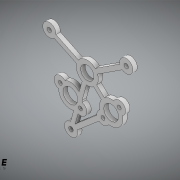
# Autodesk Inventor part: モーターマウントっぽい
Saved by Autodesk Inventor 2020 (Build 240168000, 168)
## iProperties
Created: 2020-01-28
Part Number: モーターマウントっぽい
Material: 一般
Document SubType Name: Modeling
Designer: tanjihayato
Density: 1 g/cm^3
Appearance: 既定
Author: tanjihayato
Autodesk Inventor part; units mm, degrees
ref_plane "YZ Plane" through (0, 0, 0) normal (1, 0, 0) x (0, 1, 0)
ref_plane "XZ Plane" through (0, 0, 0) normal (0, 1, 0) x (-1, 0, 0)
ref_plane "XY Plane" through (0, 0, 0) normal (0, 0, 1) x (1, 0, 0)
sketch "スケッチ1" plane through (0, 0, 0) normal (0, 0, 1) x (1, 0, 0)
  circle A0 centre (16.245, -15.3385) radius 5
  circle A1 centre (21.7373, -9.5217) radius 1.3
  circle A2 centre (10.7528, -21.1553) radius 1.3
  circle A3 centre (-4.6327, -23.2746) radius 1.3
  circle A4 centre (-11.4931, -19.1593) radius 5
  circle A5 centre (-18.3534, -15.044) radius 1.3
  circle A6 centre (26.4774, 17.2466) radius 1.5
  circle A7 centre (-11.0721, -38.6885) radius 1.5
  circle A8 centre (-25.8354, 12.3344) radius 1.5
  circle A9 centre (-11.4931, -19.1593) radius 8
  circle A10 centre (-4.6327, -23.2746) radius 4.3
  circle A11 centre (10.7528, -21.1553) radius 4.3
  circle A12 centre (16.245, -15.3385) radius 8
  circle A13 centre (21.7373, -9.5217) radius 4.3
  circle A14 centre (26.4774, 17.2466) radius 4.5
  circle A15 centre (-25.8354, 12.3344) radius 4.5
  circle A16 centre (-11.0721, -38.6885) radius 4.5
  circle A17 centre (-18.3534, -15.044) radius 4.3
  circle A18 centre (0, 0) radius 4.5
  circle A19 centre (0, 0) radius 7.5
  line L0 (-25.8354, 12.3344) -> (0, 0) construction
  line L1 (-26.4817, 10.9807) -> (-0.6463, -1.3536)
  line L2 (0.6463, 1.3536) -> (-25.1892, 13.688)
  arc A20 (-25.1892, 13.688) -> (-26.4817, 10.9807) centre (-25.8354, 12.3344) ccw
  arc A21 (-0.6463, -1.3536) -> (0.6463, 1.3536) centre (0, 0) ccw
  line L3 (26.4774, 17.2466) -> (0, 0) construction
  line L4 (25.6587, 18.5034) -> (-0.8187, 1.2569)
  line L5 (0.8187, -1.2569) -> (27.2961, 15.9897)
  arc A22 (27.2961, 15.9897) -> (25.6587, 18.5034) centre (26.4774, 17.2466) ccw
  arc A23 (-0.8187, 1.2569) -> (0.8187, -1.2569) centre (0, 0) ccw
  line L6 (0, 0) -> (-11.0721, -38.6885) construction
  line L7 (-1.4421, 0.4127) -> (-12.5142, -38.2758)
  line L8 (-9.63, -39.1013) -> (1.4421, -0.4127)
  arc A24 (1.4421, -0.4127) -> (-1.4421, 0.4127) centre (0, 0) ccw
  arc A25 (-12.5142, -38.2758) -> (-9.63, -39.1013) centre (-11.0721, -38.6885) ccw
  line L9 (0, 0) -> (16.245, -15.3385) construction
  line L10 (-1.0298, -1.0907) -> (15.2152, -16.4292)
  line L11 (17.2748, -14.2479) -> (1.0298, 1.0907)
  arc A26 (1.0298, 1.0907) -> (-1.0298, -1.0907) centre (0, 0) ccw
  arc A27 (15.2152, -16.4292) -> (17.2748, -14.2479) centre (16.245, -15.3385) ccw
  line L12 (16.245, -15.3385) -> (-11.0721, -38.6885) construction
  line L13 (15.2704, -14.1983) -> (-12.0467, -37.5483)
  line L14 (-10.0975, -39.8288) -> (17.2197, -16.4787)
  arc A28 (17.2197, -16.4787) -> (15.2704, -14.1983) centre (16.245, -15.3385) ccw
  arc A29 (-12.0467, -37.5483) -> (-10.0975, -39.8288) centre (-11.0721, -38.6885) ccw
  point P0 (-12.9177, 6.1672)
  point P1 (13.2387, 8.6233)
  point P2 (-5.5361, -19.3443)
  point P3 (8.1225, -7.6693)
  point P4 (2.5865, -27.0135)
  point P5 (17.9324, -7.5185)
  point P6 (11.5612, -8.853)
  point P7 (6.3729, -3.9543)
  point P8 (6.9761, 2.7539)
  point P9 (23.7411, 13.6741)
  point P10 (22.1037, 16.1878)
  point P11 (5.3387, 5.2676)
  point P12 (-5.9852, 4.5196)
  point P13 (-21.3605, 11.8601)
  point P14 (-22.653, 9.1528)
  point P15 (-7.2777, 1.8124)
  point P16 (-3.464, -6.6521)
  point P17 (-5.5202, -13.8372)
  point P18 (-15.2318, -12.0867)
  point P19 (-19.493, -19.1903)
  point P20 (-9.2402, -26.8356)
  point P21 (-11.3469, -34.1969)
  point P22 (-6.8724, -37.0721)
  point P23 (7.9418, -24.4093)
  point P24 (14.5577, -23.1585)
  point P25 (23.9554, -13.2054)
  point P26 (-5.4098, -24.3549)
  point P27 (-5.4008, -24.3235)
  point P28 (-5.3898, -24.3314)
  point P29 (-3.5822, -17.9687)
  point P30 (-0.5798, -7.4776)
  point P31 (4.3133, -6.1356)
  point P32 (9.5016, -11.0343)
  point P33 (8.5347, -17.4716)
  point P34 (6.4881, -21.7052)
  point P35 (-8.259, -34.3107)
  point P36 (-6.2418, -27.2622)
  point P37 (-3.4931, -19.1284)
  dimension "d0" = 3
  dimension "d1" = 3
  dimension "d2" = 3
  dimension "d3" = 3
  dimension "d4" = 3
  dimension "d5" = 3
  dimension "d6" = 3
  dimension "d7" = 3
  dimension "d8" = 3
  dimension "d9" = 9
  dimension "d10" = 3
  dimension "d11" = 3
  dimension "d12" = 3
  dimension "d13" = 3
  dimension "d14" = 3
  dimension "d15" = 3
  constraints: 40 end point, 30 centre point, 20 point on circle, 20 tangent, 5 midpoint, 5 parallel, 3 concentric, 1 coincident
  measures "d0" radial gap between concentric circles of A4 A9
  measures "d1" radial gap between concentric circles of A3 A10
  measures "d2" radial gap between concentric circles of A2 A11
  measures "d3" radial gap between concentric circles of A0 A12
  measures "d4" radial gap between concentric circles of A1 A13
  measures "d5" radial gap between concentric circles of A6 A14
  measures "d6" radial gap between concentric circles of A8 A15
  measures "d7" radial gap between concentric circles of A7 A16
  measures "d8" radial gap between concentric circles of A5 A17
  measures "d9" diameter of A18
  measures "d10" radial gap between concentric circles of A18 A19
  measures "d11" diameter of A21
  measures "d12" diameter of A23
  measures "d13" diameter of A25
  measures "d14" diameter of A27
  measures "d15" diameter of A29
extrude "押し出し1" add sketch "スケッチ1" along normal blind 3 contours A0 A13 A12 A11 | A0 A13 A12 A1 | A11 A12 A2 L14 A0 | A0 L11 A12 A13 | A12 A1 A13 | L14 A2 A12 L13 A0 | A0 L10 A12 L11 | L13 A12 A11 A0 | A11 L14 A2 A12 | A0 A11 A12 L10 | A12 L10 A19 L11 | L13 A11 A12 | A12 A2 L14 A11 L13 | L14 A16 L8 L13 A11 | L11 A18 L5 A19 | A19 L10 A18 L11 | L14 A7 L8 A16 | A16 L7 A7 L14 | A19 L8 A18 L10 | L13 A16 L7 A9 A10 L8 | L8 A16 L13 | L8 A7 L13 A16 | L8 A9 L7 A19 | A19 L7 A18 L8 | L5 A18 L4 A19 | A19 L4 A14 L5 | L8 A9 A3 A10 | A10 A9 L8 | L13 A7 L7 A16 | A19 L1 A18 L7 | L8 A10 A4 L7 A9 | A9 A10 L8 | L4 A18 L2 A19 | L5 A6 L4 A14 | A14 L4 A6 L5 | A10 L7 A4 L8 A3 A9 | A9 L7 A10 | A9 A17 A4 A10 L7 | L1 A15 L2 A19 | A19 L2 A18 L1 | L7 A4 A17 A9 | A9 A3 L8 A10 | A10 A4 L7 | A17 A9 A5 | A9 A5 A17 A4 | L1 A8 L2 A15 | A15 L2 A8 L1 picked at (-8.3681, -23.5569)
